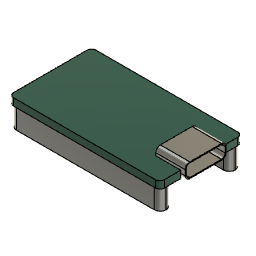
nice-nano (Autodesk Fusion 360 design; units mm, degrees)
Autodesk Fusion 360 part; units mm, degrees
note: some values were not read from the file. Set by a fixed rule: which sketch regions a step uses.
sketch "Outline" plane through (0, 0, 0) normal (0, 0, 1) x (-1, 0, 0)
  line L0 (-17.65, 4.5) -> (-11.15, 4.5)
  line L1 (-11.15, 4.5) -> (-11.15, -4.5)
  line L2 (-11.15, -4.5) -> (-17.65, -4.5)
  line L3 (-17.65, -4.5) -> (-17.65, 4.5)
  line L4 (-17.65, 4.5) -> (-11.15, -4.5) construction
  line L5 (-11.15, 4.5) -> (-17.65, -4.5) construction
  line L6 (-16.65, 9.1) -> (16.65, 9.1)
  line L7 (16.65, 9.1) -> (16.65, -9.1)
  line L8 (16.65, -9.1) -> (-16.65, -9.1)
  line L9 (-16.65, 9.1) -> (16.65, -9.1) construction
  line L10 (16.65, 9.1) -> (-16.65, -9.1) construction
  line L11 (0, 0) -> (-14.4, 0) construction
  line L12 (0, 0) -> (-14.4, 0) construction
  line L13 (-16.65, -9.1) -> (-16.65, -4.5)
  line L14 (-16.65, 4.5) -> (-16.65, 9.1)
  point P0 (16.65, 0)
  dimension "d29" = 6.5
  dimension "d30" = 9
  dimension "d31" = 33.3
  dimension "d32" = 18.2
  dimension "d33" = 1
  constraint horizontal L0
  constraint perpendicular L0 L1
  constraint parallel L0 L2
  constraint parallel L1 L3
  constraint coincident L4 L11.end
  constraint coincident L5 L11.end
  constraint horizontal L6
  constraint perpendicular L6 L7
  constraint parallel L6 L8
  constraint parallel L7 L13
  constraint coincident L9 L11.start
  constraint coincident L10 L11.start
  constraint coincident L11.start L12.start
  constraint coincident L11.end L12.end
  constraint horizontal L12
  constraint collinear L13 L14
  constraint coincident L2 L13.end
  constraint coincident L0 L14.start
  constraint midpoint L7 P0
  measures "d29" distance of L1.end L2.end
  measures "d30" distance of L0.end L1.end
  measures "d31" distance of L7.end L8.end
  measures "d32" distance of L6.start L8.end
  measures "d33" distance of L3 L13
extrude "Extrude1" add sketch "Outline" along normal blind 1.6 contours L0 L1 L2 L6 L7 L8 L13 L14 makes body 1
extrude "Extrude2" add sketch "Outline" along normal blind 3.2 separate body contours L0 L1 L2 L3 makes body 2
fillet "Fillet1" radius 1 4 edges at (14.4, -4.5, 0) (14.4, -4.5, 3.2) (14.4, 4.5, 3.2) (14.4, 4.5, 0) on bodies 2
shell "Shell1" thickness 0.2 removed faces 1 at (17.65, -1.1667, 2.1333) on bodies 2
fillet "Fillet2" radius 1 4 edges at (16.65, -9.1, 0.8) (16.65, 9.1, 0.8) (-16.65, 9.1, 0.8) (-16.65, -9.1, 0.8) on bodies 1
sketch "kaki" plane through (0, 0, 0) normal (0, 0, 1) x (-1, 0, 0)
  line L0 (16.65, 9.1) -> (16.65, -9.1)
  line L1 (-16.65, -9.1) -> (-16.65, -4.5)
  line L2 (16.65, -9.1) -> (-16.65, -9.1)
  line L3 (0, 0) -> (-14.4, 0)
  circle A0 centre (15.24, -7.62) radius 0.546
  circle A1 centre (12.7, -7.62) radius 0.546
  circle A2 centre (10.16, -7.62) radius 0.546
  circle A3 centre (7.62, -7.62) radius 0.546
  circle A4 centre (5.08, -7.62) radius 0.546
  circle A5 centre (2.54, -7.62) radius 0.546
  circle A6 centre (0, -7.62) radius 0.546
  circle A7 centre (-2.54, -7.62) radius 0.546
  circle A8 centre (-5.08, -7.62) radius 0.546
  circle A9 centre (-7.62, -7.62) radius 0.546
  circle A10 centre (-10.16, -7.62) radius 0.546
  circle A11 centre (-12.7, -7.62) radius 0.546
  circle A12 centre (-15.24, -7.62) radius 0.546
  line L4 (16.51, -8.89) -> (-16.51, -8.89)
  line L5 (-16.51, -8.89) -> (-16.51, -6.35)
  line L6 (-16.51, -6.35) -> (16.51, -6.35)
  line L7 (16.51, -6.35) -> (16.51, -8.89)
  line L8 (15.24, -7.62) -> (19.0265, -7.62) construction
  line L9 (0, -7.62) -> (0, -10.58) construction
  line L10 (-16.51, 8.89) -> (16.51, 8.89)
  line L11 (16.51, 8.89) -> (16.51, 6.35)
  line L12 (16.51, 6.35) -> (-16.51, 6.35)
  line L13 (-16.51, 6.35) -> (-16.51, 8.89)
  circle A13 centre (15.24, 7.62) radius 0.546
  circle A14 centre (12.7, 7.62) radius 0.546
  circle A15 centre (10.16, 7.62) radius 0.546
  circle A16 centre (7.62, 7.62) radius 0.546
  circle A17 centre (5.08, 7.62) radius 0.546
  circle A18 centre (2.54, 7.62) radius 0.546
  circle A19 centre (0, 7.62) radius 0.546
  circle A20 centre (-2.54, 7.62) radius 0.546
  circle A21 centre (-5.08, 7.62) radius 0.546
  circle A22 centre (-7.62, 7.62) radius 0.546
  circle A23 centre (-10.16, 7.62) radius 0.546
  circle A24 centre (-12.7, 7.62) radius 0.546
  circle A25 centre (-15.24, 7.62) radius 0.546
  line L14 (15.24, 7.62) -> (21, 7.62) construction
  line L15 (0, -7.62) -> (0, 7.62)
  point P0 (9, -12.3232)
  point P1 (16.51, -7.62)
  point P2 (16.51, 7.62)
  dimension "d23" = 2.54
  dimension "d24" = 0
  dimension "d27" = 1.092
  dimension "d28" = 2.54
  dimension "d34" = 1.27
  dimension "d35" = 1.27
  dimension "d48" = 2.54
  dimension "d49" = 0
  dimension "d50" = 1.092
  dimension "d51" = 2.54
  dimension "d52" = 15.24
  dimension "d53" = 1.27
  constraint horizontal L4
  constraint vertical L5
  constraint horizontal L6
  constraint vertical L7
  constraint midpoint L7 P1
  constraint coincident A0.centre L8.start
  constraint horizontal L8
  constraint coincident P1 L8
  constraint coincident A6.centre L9.start
  constraint perpendicular L4 L9
  constraint midpoint L2 L9
  constraint horizontal L12
  constraint vertical L13
  constraint horizontal L10
  constraint vertical L11
  constraint coincident A13.centre L14.start
  constraint parallel L10 L14
  constraint midpoint L11 P2
  constraint coincident L14 P2
  constraint collinear L7 L11
  constraint coincident A19.centre L15.end
  constraint midpoint L15 L3.start
  constraint coincident L3 origin
  measures "d27" diameter of A0
  measures "d28" distance of L4.start L6.end
  measures "d34" distance of A0.centre L7
  measures "d35" distance of A12.centre L5
  measures "d50" diameter of A13
  measures "d51" distance of L11.end L10.end
  measures "d52" distance of A0.centre A13.centre
  measures "d53" distance of A13.centre P2
extrude "Extrude3" add sketch "kaki" against normal blind 4.5 separate body makes body 3 at (-5.5033, 8.89, -1.5) makes body 4 at (5.5033, -8.89, -1.5)
fillet "Fillet3" radius 1.3 8 edges at (16.51, 6.35, -2.25) (16.51, 8.89, -2.25) (-16.51, 6.35, -2.25) (-16.51, 8.89, -2.25) (-16.51, -8.89, -2.25) (-16.51, -6.35, -2.25) (16.51, -8.89, -2.25) (16.51, -6.35, -2.25) on bodies 3 4
equation "d31 = nn_length"
equation "d32 = nn_width"
equation "d37 = nn_thickness"
equation "d39 = nn_usb_thickness"
equation "d111 = tc_z_offset"
equation "d112 = tc_y_offset"
equation "d113 = tc_x_offset"
equation "nn_width = 18.2 mm"
equation "nn_length = 33.3 mm"
equation "nn_thickness = 1.6 mm"
equation "nn_usb_thickness = 3.2 mm"
equation "tc_x_offset = 4 mm"
equation "tc_y_offset = 1 mm"
equation "tc_z_offset = 1 mm"
equation "nn_clearance = 4.5 mm"
equation "d5 = -nn_clearance"
equation "nn_hole_pitch = 2.54 mm"
equation "d28 = nn_hole_pitch"
equation "d34 = nn_hole_pitch / 2"
equation "d35 = d34"
equation "d51 = nn_hole_pitch"
equation "d53 = d34"
named bodies: "Pcb", "Connector"
